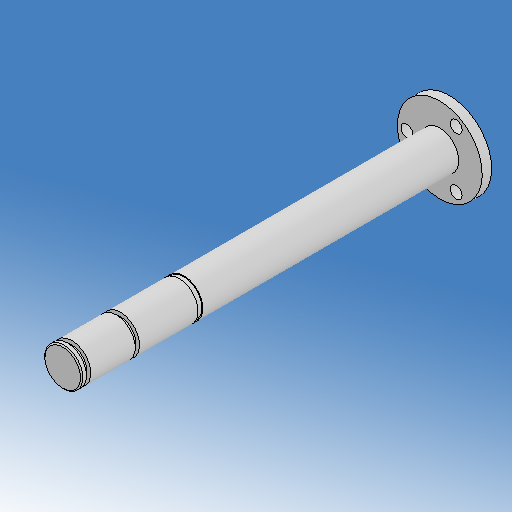
# Autodesk Inventor part: FlipperH5055RoundShaft
Saved by Autodesk Inventor 2025 (Build 290162000, 162)
## iProperties
Created: 2024-02-07
Part Number: FlipperH5055RoundShaft
Material: Generic
Document SubType Name: Modeling
Designer: seene
Density: 1 g/cm^3
Appearance: Default
Author: seene
Autodesk Inventor part; units mm, degrees
ref_plane "YZ Plane" through (0, 0, 0) normal (1, 0, 0) x (0, 1, 0)
ref_plane "XZ Plane" through (0, 0, 0) normal (0, 1, 0) x (-1, 0, 0)
ref_plane "XY Plane" through (0, 0, 0) normal (0, 0, 1) x (1, 0, 0)
sketch "Sketch2" plane through (0, 0, 0) normal (1, 0, 0) x (0, 1, 0)
  line L0 (0, 0) -> (-3.985, 0)
  line L1 (0, -80.84) -> (0.015, -80.84)
  line L2 (-8.87, -80.84) -> (0, -80.84)
  line L3 (-3.985, -78.84) -> (-8.87, -78.84)
  line L4 (-8.87, -78.84) -> (-8.87, -80.84)
  line L5 (-3.985, -24.34) -> (-3.785, -24.34)
  line L6 (-3.785, -24.34) -> (-3.785, -25.34)
  line L7 (-3.785, -25.34) -> (-3.985, -25.34)
  line L8 (-3.985, -25.34) -> (-3.985, -24.34)
  line L9 (0, 0) -> (0, -80.84)
  line L10 (-6.435, 0) -> (-6.435, -12.64) construction
  line L11 (-6.435, -12.64) -> (0, -12.64) construction
  line L12 (-3.985, 0) -> (-3.985, -24.34)
  line L13 (-3.985, -25.34) -> (-3.985, -78.84)
  line L14 (0, 0) -> (0, -80.84)
  line L15 (-3.985, -1) -> (-3.185, -1)
  line L16 (-3.185, -1) -> (-3.185, -1.9)
  line L17 (-3.185, -1.9) -> (-3.985, -1.9)
  line L18 (-3.985, -1.9) -> (-3.985, -1)
  line L19 (2.8591, -2.1) -> (-4.9211, -2.1) construction
  line L20 (-4.9211, -2.1) -> (-4.9211, -10.99) construction
  line L21 (-4.9211, -10.99) -> (2.8591, -10.99) construction
  line L22 (2.8591, -10.99) -> (2.8591, -2.1) construction
  line L23 (-3.985, -11.19) -> (-3.185, -11.19)
  line L24 (-3.185, -11.19) -> (-3.185, -12.09)
  line L25 (-3.185, -12.09) -> (-3.985, -12.09)
  line L26 (-3.985, -12.09) -> (-3.985, -11.19)
  point P0 (-8.87, -79.84)
  point P1 (-4.9211, -6.545)
  point P2 (-3.585, -1)
  point P3 (-3.985, -12.09)
  dimension "d3" = 1
  dimension "d5" = 0.2
  dimension "d18" = 55.5
  dimension "d21" = 2
  dimension "d22" = 17.74
  dimension "d24" = 12.64
  dimension "d25" = 6.435
  dimension "d26" = 12.7
  dimension "d35" = 0.9
  dimension "d36" = 0.8
  dimension "d38" = 8.89
  dimension "d39" = 0.2
  dimension "d40" = 1
  dimension "d41" = 3.985
  dimension "d45" = 0.2
  constraints: 54 end point, 10 parallel, 7 horizontal, 6 perpendicular, 4 vertical, 3 midpoint, 3 point on line, 2 coincident, 2 equal length, 1 horizontal alignment
  measures "d3" distance of L5.end L6.end
  measures "d5" distance of L6.end L7.end
  measures "d18" distance between parallel lines of L2 L7
  measures "d21" distance between parallel lines of L2 L3
  measures "d22" diameter of L4 L9
  measures "d24" distance of L10.start L10.end
  measures "d25" distance of L10.end L11.end
  measures "d26" distance between parallel lines of L11 L7
  measures "d35" distance of L15.end L16.end
  measures "d36" distance of L16.end L17.end
  measures "d38" distance between parallel lines of L21 L19
  measures "d39" distance between parallel lines of L19 L17
  measures "d40" distance from line of point (-3.585, -1) L0
  measures "d41" distance of L0.start L0.end
  measures "d45" distance between parallel lines of L23 L21
revolve "Revolution1" add sketch "Sketch2" angle 360 about axis through (0, 0, 0) along (0, 0, -1) contours L9 L2 L4 L3 L13 L7 L6 L5 L12 L25 L24 L23 L17 L16 L15 L0
sketch "Sketch4" plane through (0, 0, -80.84) normal (0, 0, -1) x (-1, 0, 0)
  circle A0 centre (0, 0) radius 6.87 construction
  circle A1 centre (6.87, 0) radius 1.25
  circle A2 centre (0, 0) radius 8.87 projected
  circle A3 centre (-3.435, 5.9496) radius 1.25
  circle A4 centre (-3.435, -5.9496) radius 1.25
  dimension "d28" = 2.5
  dimension "d46" = 2
  dimension "d49" = 360
  constraints: 3 centre point, 2 horizontal alignment, 1 coincident, 9 other
  measures "d28" diameter of A1
extrude "Extrusion2" cut sketch "Sketch4" against normal through all contours A1 | A3 | A4
chamfer "Chamfer1" distance 0.25 angle 45 1 edges at (0, 3.985, 0)
equation "\"d45\" = d39"
body "Solid1"
